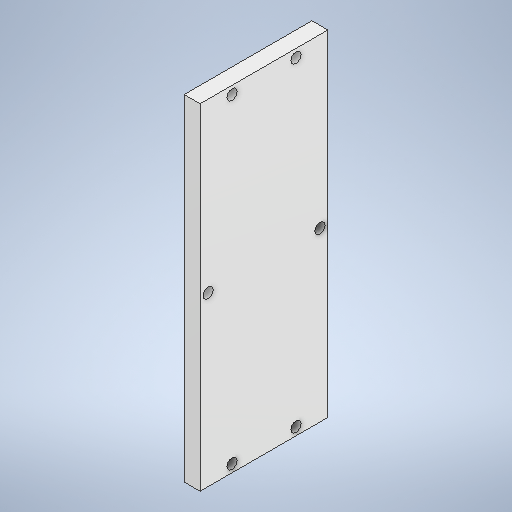
# Autodesk Inventor part: Handle_Side_Covers
Saved by Autodesk Inventor 2026.2 (Build 302298010, 298A)
## iProperties
Created: 2026-04-30
Part Number: Handle_Side_Covers
Material: ABS Plastic
Document SubType Name: Modeling
Designer: piete
Density: 1.06 g/cm^3
Appearance: Smooth - White
Author: piete
Autodesk Inventor part; units mm, degrees
ref_plane "YZ Plane" through (0, 0, 0) normal (1, 0, 0) x (0, 1, 0)
ref_plane "XZ Plane" through (0, 0, 0) normal (0, 1, 0) x (-1, 0, 0)
ref_plane "XY Plane" through (0, 0, 0) normal (0, 0, 1) x (1, 0, 0)
sketch "Sketch1" plane through (0, 0, 0) normal (1, 0, 0) x (0, 1, 0)
  line L0 (52.5, 20) -> (-52.5, 20)
  line L1 (-52.5, 20) -> (-52.5, -20)
  line L2 (-52.5, -20) -> (52.5, -20)
  line L3 (52.5, -20) -> (52.5, 20)
  circle A0 centre (50, 10) radius 1.6
  circle A1 centre (0, 17.5) radius 1.6
  circle A2 centre (50, -10) radius 1.6
  circle A3 centre (0, -17.5) radius 1.6
  circle A4 centre (-50, 10) radius 1.6
  circle A5 centre (-50, -10) radius 1.6
  point P0 (0, 0)
  point P1 (52.5, 0)
  point P2 (-52.5, 0)
  dimension "d0" = 105
  dimension "d1" = 40
  dimension "d2" = 52.5
  dimension "d3" = 20
  dimension "d4" = 3.2
  dimension "d5" = 3.2
  dimension "d6" = 3.2
  dimension "d7" = 3.2
  dimension "d8" = 3.2
  dimension "d9" = 3.2
  dimension "d10" = 2.5
  dimension "d11" = 2.5
  dimension "d12" = 10
  dimension "d13" = 10
  dimension "d14" = 0
  dimension "d15" = 2.5
  dimension "d16" = 2.5
  dimension "d17" = 0
  dimension "d18" = 2.5
  dimension "d19" = 2.5
  dimension "d20" = 10
  dimension "d21" = 10
  constraints: 8 end point, 6 centre point, 2 midpoint, 2 parallel, 1 horizontal, 1 perpendicular
  measures "d0" distance of L2.end L1.end
  measures "d1" distance of L1.end L0.end
  measures "d2" distance from line of L3 point (0, 0)
  measures "d3" distance from line of L0 point (0, 0)
  measures "d4" diameter of A0
  measures "d5" diameter of A1
  measures "d6" diameter of A2
  measures "d7" diameter of A3
  measures "d8" diameter of A4
  measures "d9" diameter of A5
  measures "d10" distance from line of L3 A0.centre
  measures "d11" distance from line of L3 A2.centre
  measures "d12" vertical distance of point (52.5, 0) A2.centre
  measures "d13" vertical distance of point (52.5, 0) A0.centre
  measures "d14" horizontal distance of point (0, 0) A1.centre
  measures "d15" distance from line of L0 A1.centre
  measures "d16" distance from line of L2 A3.centre
  measures "d17" horizontal distance of point (0, 0) A3.centre
  measures "d18" distance from line of L1 A4.centre
  measures "d19" distance from line of L1 A5.centre
  measures "d20" vertical distance of point (-52.5, 0) A5.centre
  measures "d21" vertical distance of point (-52.5, 0) A4.centre
extrude "Extrusion1" add sketch "Sketch1" along normal blind 5
equation "\"d2\" = 0.5 * d0"
equation "\"d3\" = 0.5 * d1"
body "Solid1"
